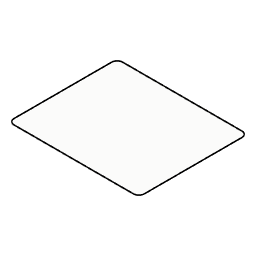
Deskpad-V1 (Autodesk Fusion 360 design; units mm, degrees)
Autodesk Fusion 360 part; units mm, degrees
sketch "Skizze1" plane through (0, 0, 0) normal (0, 0, 1) x (1, 0, 0)
  line L0 (125, 150) -> (1225, 150)
  line L1 (1275, 100) -> (1275, -800)
  line L2 (1225, -850) -> (125, -850)
  line L3 (75, -800) -> (75, 100)
  arc A0 (125, 150) -> (75, 100) centre (125, 100) ccw
  arc A1 (1275, 100) -> (1225, 150) centre (1225, 100) ccw
  arc A2 (1225, -850) -> (1275, -800) centre (1225, -800) ccw
  arc A3 (75, -800) -> (125, -850) centre (125, -800) ccw
  point P0 (75, 150)
  point P1 (1275, 150)
  point P2 (75, -850)
  dimension "d1" = 1200
  dimension "d2" = 1000
  dimension "d3" = 50
  dimension "d4" = 50
  constraint horizontal L0
  constraint vertical L1
  constraint horizontal L2
  constraint vertical L3
  constraint coincident P0 L0
  constraint coincident P0 L3
  constraint tangent L0 A0
  constraint tangent L3 A0
  constraint coincident P1 L0
  constraint coincident P1 L1
  constraint tangent L0 A1
  constraint tangent L1 A1
  constraint equal A0 A1
  constraint tangent L1 A2
  constraint tangent L2 A2
  constraint equal A0 A2
  constraint coincident P2 L2
  constraint coincident P2 L3
  constraint tangent L2 A3
  constraint tangent L3 A3
  measures "d1" distance of P0 P1
  measures "d2" distance of P0 P2
  measures "d3" radius of A0
  measures "d4" radius of A3
extrude "Extrusion1" add sketch "Skizze1" along normal blind 2
equation "d4 = d3"
named bodies: "body"
